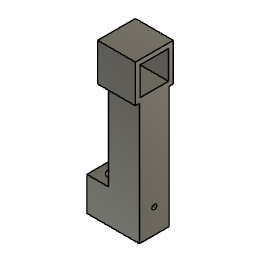
Arm Part v1 (Autodesk Fusion 360 design; units mm, degrees)
Autodesk Fusion 360 part; units mm, degrees
note: some values were not read from the file. Set by a fixed rule: which sketch regions a step uses.
sketch "Sketch1" plane through (0, 0, 0) normal (0, 0, 1) x (1, 0, 0)
  circle A0 centre (0, 0) radius 6.604
  line L0 (-12.827, 13.97) -> (36.703, 13.97)
  line L1 (36.703, 13.97) -> (36.703, -13.97)
  line L2 (36.703, -13.97) -> (-12.827, -13.97)
  line L3 (-12.827, -13.97) -> (-12.827, 13.97)
  line L4 (16.129, 10.287) -> (31.623, 10.287)
  line L5 (31.623, 10.287) -> (31.623, -10.287)
  line L6 (31.623, -10.287) -> (16.129, -10.287)
  line L7 (16.129, -10.287) -> (16.129, 10.287)
  line L8 (16.129, 0) -> (31.623, 0)
  point P0 (16.129, 0)
  point P1 (31.623, 0)
  point P2 (-12.827, 0)
  point P3 (36.703, 0)
  point P4 (23.876, 0)
  dimension "d1" = 13.208
  dimension "d2" = 15.494
  dimension "d3" = 20.574
  dimension "d4" = 23.876
  dimension "d5" = 5.08
  dimension "d6" = 49.53
  dimension "d7" = 27.94
  constraint coincident A0.centre origin
  constraint horizontal L0
  constraint vertical L1
  constraint horizontal L2
  constraint vertical L3
  constraint horizontal L4
  constraint vertical L5
  constraint horizontal L6
  constraint vertical L7
  constraint coincident L7 P0
  constraint coincident L5 P1
  constraint midpoint L7 P0
  constraint midpoint L5 P1
  constraint coincident L3 P2
  constraint coincident L1 P3
  constraint midpoint L3 P2
  constraint midpoint L1 P3
  constraint horizontal A0.centre P2
  constraint horizontal P1 P3
  constraint coincident P0 L8.start
  constraint coincident P1 L8.end
  constraint midpoint P4 L8
  measures "d1" diameter of A0
  measures "d2" distance of L5 L7
  measures "d3" distance of L4.end L5.end
  measures "d4" distance of A0.centre P4
  measures "d5" distance of L1 L5
  measures "d6" distance of L1 L3
  measures "d7" distance of L0 L2
extrude "Extrude1" add sketch "Sketch1" along normal blind 31.75
sketch "Sketch2" plane through (36.703, 0, 0) normal (1, 0, 0) x (0, 1, 0)
  line L0 (-13.97, 0) -> (13.97, 0)
  line L1 (13.97, 0) -> (13.97, 31.75)
  line L2 (13.97, 31.75) -> (-13.97, 31.75)
  line L3 (-13.97, 31.75) -> (-13.97, 0)
  line L4 (0, 0) -> (0, 40.147)
  circle A0 centre (0, 22.86) radius 2.286
  point P0 (0, 22.86)
  dimension "d10" = 8.89
  dimension "d11" = 4.572
  constraint coincident L4.start origin
  constraint perpendicular L2 L4
  constraint coincident L4 P0
  constraint coincident P0 A0.centre
  measures "d10" distance of L2 P0
  measures "d11" diameter of A0
extrude "Extrude2" cut sketch "Sketch2" against normal blind 7.62 contours L4 A0 | L4 A0
sketch "Sketch3" plane through (0, 0, 31.75) normal (0, 0, 1) x (-1, 0, 0)
  line L0 (-31.623, 10.287) -> (-16.129, 10.287)
  line L1 (-16.129, 10.287) -> (-16.129, -10.287)
  line L2 (-16.129, -10.287) -> (-31.623, -10.287)
  line L3 (-31.623, -10.287) -> (-31.623, 10.287)
  circle A0 centre (0, 0) radius 6.604
  line L4 (12.827, 13.97) -> (-36.703, 13.97)
  line L5 (-36.703, 13.97) -> (-36.703, -13.97)
  line L6 (-36.703, -13.97) -> (12.827, -13.97)
  line L7 (12.827, -13.97) -> (12.827, 13.97)
  line L8 (-7.493, -13.97) -> (-36.703, -13.97)
  line L9 (-36.703, -13.97) -> (-36.703, 13.97)
  line L10 (-36.703, 13.97) -> (-7.493, 13.97)
  line L11 (-7.493, 13.97) -> (-7.493, -13.97)
  dimension "d14" = 29.21
  constraint horizontal L8
  constraint vertical L9
  constraint horizontal L10
  constraint vertical L11
  constraint coincident L4.end L5.start
  constraint coincident L6 L8.start
  measures "d14" distance of L9 L11
extrude "Extrude3" add sketch "Sketch3" along normal blind 82.55 contours L0 L1 L2 L3 | L4 L5 L6 L8 L9 L10 L11
sketch "Sketch4" plane through (0, 0, 114.3) normal (0, 0, 1) x (-1, 0, 0)
  line L0 (-7.493, 13.97) -> (-36.703, 13.97)
  line L1 (-36.703, 13.97) -> (-36.703, -13.97)
  line L2 (-36.703, -13.97) -> (-7.493, -13.97)
  line L3 (-7.493, -13.97) -> (-7.493, 13.97)
  line L4 (-36.703, -17.78) -> (-1.143, -17.78)
  line L5 (-1.143, -17.78) -> (-1.143, 17.78)
  line L6 (-1.143, 17.78) -> (-36.703, 17.78)
  line L7 (-36.703, 17.78) -> (-36.703, -17.78)
  line L8 (-36.703, -17.78) -> (-1.143, 17.78) construction
  line L9 (-1.143, -17.78) -> (-36.703, 17.78) construction
  line L10 (-36.703, -13.97) -> (-36.703, 13.97)
  point P0 (-18.923, 0)
  dimension "d17" = 35.56
  dimension "d18" = 35.56
  constraint horizontal L4
  constraint perpendicular L4 L5
  constraint parallel L4 L6
  constraint parallel L5 L7
  constraint coincident L8 P0
  constraint coincident L9 P0
  constraint horizontal origin P0
  constraint coincident L1.end L2.start
  constraint coincident L0.end L1.start
  constraint collinear L7 L10
  measures "d17" distance of L5 L7
  measures "d18" distance of L4.start L6.end
extrude "Extrude4" add sketch "Sketch4" along normal blind 35.56
sketch "Sketch5" plane through (36.703, 0, 0) normal (1, 0, 0) x (0, 1, 0)
  circle A0 centre (0, 22.86) radius 2.286
  line L0 (-13.97, 0) -> (13.97, 0)
  line L1 (13.97, 0) -> (13.97, 114.3)
  line L2 (13.97, 114.3) -> (17.78, 114.3)
  line L3 (17.78, 114.3) -> (17.78, 149.86)
  line L4 (17.78, 149.86) -> (-17.78, 149.86)
  line L5 (-17.78, 149.86) -> (-17.78, 114.3)
  line L6 (-17.78, 114.3) -> (-13.97, 114.3)
  line L7 (-13.97, 114.3) -> (-13.97, 0)
  line L8 (-13.335, 145.415) -> (13.335, 145.415)
  line L9 (13.335, 145.415) -> (13.335, 118.745)
  line L10 (13.335, 118.745) -> (-13.335, 118.745)
  line L11 (-13.335, 118.745) -> (-13.335, 145.415)
  dimension "d21" = 4.445
  dimension "d22" = 4.445
  dimension "d23" = 4.445
  dimension "d24" = 4.445
  constraint horizontal L8
  constraint vertical L9
  constraint horizontal L10
  constraint vertical L11
  measures "d21" distance of L5.end L10
  measures "d22" distance of L4 L8
  measures "d23" distance of L5 L11
  measures "d24" distance of L3 L9
extrude "Extrude5" cut sketch "Sketch5" against normal blind 45.72 contours L8 L9 L10 L11
